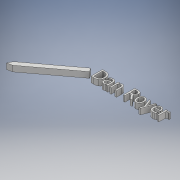
# Autodesk Inventor part: dan2
Saved by Autodesk Inventor 2017 (Build 210142000, 142)
## iProperties
Created: 2021-02-26
Part Number: dan2
Material: Generic
Document SubType Name: Modeling
Designer: paulg
Density: 1 g/cm^3
Appearance: Default
Author: paulg
Autodesk Inventor part; units mm, degrees
ref_plane "YZ Plane" through (0, 0, 0) normal (1, 0, 0) x (0, 1, 0)
ref_plane "XZ Plane" through (0, 0, 0) normal (0, 1, 0) x (-1, 0, 0)
ref_plane "XY Plane" through (0, 0, 0) normal (0, 0, 1) x (1, 0, 0)
sketch "Sketch1" plane through (0, 0, 0) normal (0, 0, 1) x (1, 0, 0)
  line L0 (-0.0217, 0.1086) -> (142.61, 0.1086) construction
  line L1 (142.61, 0.1086) -> (142.61, -1.7562) construction
  line L2 (142.61, -1.7562) -> (-0.0217, -1.7562) construction
  line L3 (-0.0217, -1.7562) -> (-0.0217, 0.1086) construction
  line L4 (-41.7116, -36.1087) -> (-2.9577, -7.16)
  line L5 (-2.9577, -7.16) -> (-5.3043, -4.0186)
  line L6 (-5.3043, -4.0186) -> (-44.0582, -32.9673)
  line L7 (-44.0582, -32.9673) -> (-41.7116, -36.1087)
  line L8 (-41.7116, -36.1087) -> (-5.3043, -4.0186) construction
  line L9 (-2.9577, -7.16) -> (-44.0582, -32.9673) construction
  line L10 (-44.0582, -32.9673) -> (-46.1916, -37.008)
  line L11 (-46.1916, -37.008) -> (-41.7116, -36.1087)
  line L12 (-46.1916, -37.008) -> (-42.8849, -34.538) construction
  spline S0 degree 2 poles (8.8762, -4.8995) (8.8762, -6.269) (7.766, -8.4732) (6.834, -9.0891) knots 0 0 0 1 2 2 2
  spline S1 degree 2 poles (6.834, -9.0891) (6.0723, -9.5672) (4.5083, -9.8914) (3.2927, -9.8914) knots 0 0 0 1 2 2 2
  line L13 (3.2927, -9.8914) -> (0.9912, -9.8914)
  line L14 (0.9912, -9.8914) -> (0.9912, 0.1086)
  line L15 (0.9912, 0.1086) -> (3.2684, 0.1086)
  spline S2 degree 2 poles (3.2684, 0.1086) (4.6784, 0.1086) (6.283, -0.3127) (6.8502, -0.6855) knots 0 0 0 1 2 2 2
  spline S3 degree 2 poles (6.8502, -0.6855) (7.8146, -1.3257) (8.8762, -3.4408) (8.8762, -4.8995) knots 0 0 0 1 2 2 2
  spline S4 degree 2 poles (7.4904, -4.8833) (7.4904, -3.7325) (6.7287, -2.1037) (5.975, -1.6418) knots 0 0 0 1 2 2 2
  spline S5 degree 2 poles (5.975, -1.6418) (5.4402, -1.3257) (4.2327, -1.0421) (3.3332, -1.0421) knots 0 0 0 1 2 2 2
  line L16 (3.3332, -1.0421) -> (2.3202, -1.0421)
  line L17 (2.3202, -1.0421) -> (2.3202, -8.7406)
  line L18 (2.3202, -8.7406) -> (3.3332, -8.7406)
  spline S6 degree 2 poles (3.3332, -8.7406) (4.2165, -8.7406) (5.5536, -8.457) (6.0966, -8.0761) knots 0 0 0 1 2 2 2
  spline S7 degree 2 poles (6.0966, -8.0761) (6.7935, -7.6061) (7.4904, -6.0502) (7.4904, -4.8833) knots 0 0 0 1 2 2 2
  spline S8 degree 2 poles (14.4029, -9.0972) (14.2489, -9.2106) (13.7303, -9.6158) (13.4872, -9.7374) knots 0 0 0 1 2 2 2
  spline S9 degree 2 poles (13.4872, -9.7374) (13.1549, -9.9157) (12.5309, -10.1021) (11.9637, -10.1021) knots 0 0 0 1 2 2 2
  spline S10 degree 2 poles (11.9637, -10.1021) (11.5018, -10.1021) (10.6671, -9.7536) (10.351, -9.4375) knots 0 0 0 1 2 2 2
  spline S11 degree 2 poles (10.351, -9.4375) (10.0512, -9.1296) (9.6865, -8.222) (9.6865, -7.7196) knots 0 0 0 1 2 2 2
  spline S12 degree 2 poles (9.6865, -7.7196) (9.6865, -6.9416) (10.3429, -5.8395) (11.0561, -5.5234) knots 0 0 0 1 2 2 2
  spline S13 degree 2 poles (11.0561, -5.5234) (11.6882, -5.2317) (13.4061, -5.0129) (14.4029, -4.9562) knots 0 0 0 1 2 2 2
  line L19 (14.4029, -4.9562) -> (14.4029, -4.7131)
  spline S14 degree 2 poles (14.4029, -4.7131) (14.4029, -4.2755) (14.1355, -3.7325) (13.8924, -3.5786) knots 0 0 0 1 2 2 2
  spline S15 degree 2 poles (13.8924, -3.5786) (13.6493, -3.4246) (12.9523, -3.3273) (12.5796, -3.3273) knots 0 0 0 1 2 2 2
  spline S16 degree 2 poles (12.5796, -3.3273) (12.142, -3.3273) (10.9588, -3.5867) (10.3672, -3.8379) knots 0 0 0 1 2 2 2
  line L20 (10.3672, -3.8379) -> (10.2943, -3.8379)
  line L21 (10.2943, -3.8379) -> (10.2943, -2.5494)
  spline S17 degree 2 poles (10.2943, -2.5494) (10.6428, -2.4521) (11.9475, -2.209) (12.5877, -2.209) knots 0 0 0 1 2 2 2
  spline S18 degree 2 poles (12.5877, -2.209) (13.3656, -2.209) (14.4272, -2.4521) (14.8486, -2.7682) knots 0 0 0 1 2 2 2
  spline S19 degree 2 poles (14.8486, -2.7682) (15.2619, -3.0761) (15.6671, -4.0567) (15.6671, -4.7617) knots 0 0 0 1 2 2 2
  line L22 (15.6671, -4.7617) -> (15.6671, -9.8914)
  line L23 (15.6671, -9.8914) -> (14.4029, -9.8914)
  line L24 (14.4029, -9.8914) -> (14.4029, -9.0972)
  line L25 (14.4029, -8.0437) -> (14.4029, -5.961)
  spline S20 degree 2 poles (14.4029, -5.961) (13.9491, -6.0016) (12.5796, -6.1393) (12.1501, -6.269) knots 0 0 0 1 2 2 2
  spline S21 degree 2 poles (12.1501, -6.269) (11.6476, -6.423) (10.9912, -7.0632) (10.9912, -7.6304) knots 0 0 0 1 2 2 2
  spline S22 degree 2 poles (10.9912, -7.6304) (10.9912, -8.2787) (11.7206, -8.9351) (12.4175, -8.9351) knots 0 0 0 1 2 2 2
  spline S23 degree 2 poles (12.4175, -8.9351) (13.0091, -8.9351) (13.9815, -8.4246) (14.4029, -8.0437) knots 0 0 0 1 2 2 2
  line L26 (23.3332, -9.8914) -> (22.069, -9.8914)
  line L27 (22.069, -9.8914) -> (22.069, -5.6126)
  spline S24 degree 2 poles (22.069, -5.6126) (22.069, -5.0939) (21.9718, -4.2025) (21.8259, -3.9351) knots 0 0 0 1 2 2 2
  spline S25 degree 2 poles (21.8259, -3.9351) (21.672, -3.6515) (21.1209, -3.376) (20.6509, -3.376) knots 0 0 0 1 2 2 2
  spline S26 degree 2 poles (20.6509, -3.376) (20.1809, -3.376) (19.1841, -3.8784) (18.706, -4.2836) knots 0 0 0 1 2 2 2
  line L28 (18.706, -4.2836) -> (18.706, -9.8914)
  line L29 (18.706, -9.8914) -> (17.4418, -9.8914)
  line L30 (17.4418, -9.8914) -> (17.4418, -2.3873)
  line L31 (17.4418, -2.3873) -> (18.706, -2.3873)
  line L32 (18.706, -2.3873) -> (18.706, -3.222)
  spline S27 degree 2 poles (18.706, -3.222) (19.2732, -2.7115) (20.3672, -2.1766) (20.9831, -2.1766) knots 0 0 0 1 2 2 2
  spline S28 degree 2 poles (20.9831, -2.1766) (22.0852, -2.1766) (23.3332, -3.6353) (23.3332, -5.021) knots 0 0 0 1 2 2 2
  line L33 (23.3332, -5.021) -> (23.3332, -9.8914)
  line L34 (37.2392, -9.8914) -> (35.5131, -9.8914)
  line L35 (35.5131, -9.8914) -> (32.3527, -5.9124)
  line L36 (32.3527, -5.9124) -> (30.8292, -5.9124)
  line L37 (30.8292, -5.9124) -> (30.8292, -9.8914)
  line L38 (30.8292, -9.8914) -> (29.5002, -9.8914)
  line L39 (29.5002, -9.8914) -> (29.5002, 0.1086)
  line L40 (29.5002, 0.1086) -> (32.0771, 0.1086)
  spline S29 degree 2 poles (32.0771, 0.1086) (32.9361, 0.1086) (34.095, -0.0777) (34.6217, -0.4181) knots 0 0 0 1 2 2 2
  spline S30 degree 2 poles (34.6217, -0.4181) (35.1484, -0.7585) (35.7562, -1.82) (35.7562, -2.6061) knots 0 0 0 1 2 2 2
  spline S31 degree 2 poles (35.7562, -2.6061) (35.7562, -3.7001) (34.6379, -5.1831) (33.6817, -5.5397) knots 0 0 0 1 2 2 2
  line L41 (33.6817, -5.5397) -> (37.2392, -9.8914)
  spline S32 degree 2 poles (34.3705, -2.7115) (34.3705, -2.2739) (34.0625, -1.6012) (33.7384, -1.3824) knots 0 0 0 1 2 2 2
  spline S33 degree 2 poles (33.7384, -1.3824) (33.4548, -1.1961) (32.7011, -1.0421) (32.1501, -1.0421) knots 0 0 0 1 2 2 2
  line L42 (32.1501, -1.0421) -> (30.8292, -1.0421)
  line L43 (30.8292, -1.0421) -> (30.8292, -4.8022)
  line L44 (30.8292, -4.8022) -> (31.9961, -4.8022)
  spline S34 degree 2 poles (31.9961, -4.8022) (32.5715, -4.8022) (33.4872, -4.5996) (33.8032, -4.2836) knots 0 0 0 1 2 2 2
  spline S35 degree 2 poles (33.8032, -4.2836) (34.095, -4.008) (34.3705, -3.2301) (34.3705, -2.7115) knots 0 0 0 1 2 2 2
  spline S36 degree 2 poles (44.1031, -6.1393) (44.1031, -8.0356) (42.2797, -10.1021) (40.7562, -10.1021) knots 0 0 0 1 2 2 2
  spline S37 degree 2 poles (40.7562, -10.1021) (39.1922, -10.1021) (37.4013, -7.9708) (37.4013, -6.1393) knots 0 0 0 1 2 2 2
  spline S38 degree 2 poles (37.4013, -6.1393) (37.4013, -4.2593) (39.2489, -2.1766) (40.7562, -2.1766) knots 0 0 0 1 2 2 2
  spline S39 degree 2 poles (40.7562, -2.1766) (42.2797, -2.1766) (44.1031, -4.2512) (44.1031, -6.1393) knots 0 0 0 1 2 2 2
  spline S40 degree 2 poles (42.7984, -6.1393) (42.7984, -4.6807) (41.7368, -3.2625) (40.7562, -3.2625) knots 0 0 0 1 2 2 2
  spline S41 degree 2 poles (40.7562, -3.2625) (39.7757, -3.2625) (38.706, -4.6807) (38.706, -6.1393) knots 0 0 0 1 2 2 2
  spline S42 degree 2 poles (38.706, -6.1393) (38.706, -7.5575) (39.7757, -9.0162) (40.7562, -9.0162) knots 0 0 0 1 2 2 2
  spline S43 degree 2 poles (40.7562, -9.0162) (41.7287, -9.0162) (42.7984, -7.5818) (42.7984, -6.1393) knots 0 0 0 1 2 2 2
  line L45 (51.2911, -2.3873) -> (47.2554, -12.6547)
  line L46 (47.2554, -12.6547) -> (45.9021, -12.6547)
  line L47 (45.9021, -12.6547) -> (47.2473, -9.5267)
  line L48 (47.2473, -9.5267) -> (44.5245, -2.3873)
  line L49 (44.5245, -2.3873) -> (45.8859, -2.3873)
  line L50 (45.8859, -2.3873) -> (47.9361, -7.9465)
  line L51 (47.9361, -7.9465) -> (49.9783, -2.3873)
  line L52 (49.9783, -2.3873) -> (51.2911, -2.3873)
  spline S44 degree 2 poles (55.505, -10.0615) (53.706, -10.0615) (51.7287, -8.0437) (51.7287, -6.1798) knots 0 0 0 1 2 2 2
  spline S45 degree 2 poles (51.7287, -6.1798) (51.7287, -4.3484) (53.6493, -2.1766) (55.1971, -2.1766) knots 0 0 0 1 2 2 2
  spline S46 degree 2 poles (55.1971, -2.1766) (55.894, -2.1766) (56.9718, -2.5818) (57.3689, -3.0113) knots 0 0 0 1 2 2 2
  spline S47 degree 2 poles (57.3689, -3.0113) (57.7741, -3.4408) (58.2036, -4.6807) (58.2036, -5.5802) knots 0 0 0 1 2 2 2
  line L53 (58.2036, -5.5802) -> (58.2036, -6.269)
  line L54 (58.2036, -6.269) -> (53.0091, -6.269)
  spline S48 degree 2 poles (53.0091, -6.269) (53.0091, -7.5737) (54.3219, -8.9594) (55.4888, -8.9594) knots 0 0 0 1 2 2 2
  spline S49 degree 2 poles (55.4888, -8.9594) (55.9021, -8.9594) (56.7044, -8.773) (57.0285, -8.6272) knots 0 0 0 1 2 2 2
  spline S50 degree 2 poles (57.0285, -8.6272) (57.3689, -8.4651) (57.8389, -8.1815) (57.9929, -8.0518) knots 0 0 0 1 2 2 2
  line L55 (57.9929, -8.0518) -> (58.0658, -8.0518)
  line L56 (58.0658, -8.0518) -> (58.0658, -9.4294)
  spline S51 degree 2 poles (58.0658, -9.4294) (57.847, -9.5186) (57.1825, -9.7779) (56.9232, -9.8508) knots 0 0 0 1 2 2 2
  spline S52 degree 2 poles (56.9232, -9.8508) (56.5585, -9.9562) (55.9588, -10.0615) (55.505, -10.0615) knots 0 0 0 1 2 2 2
  spline S53 degree 2 poles (56.9718, -5.3046) (56.9556, -4.7941) (56.7449, -4.0486) (56.5423, -3.7974) knots 0 0 0 1 2 2 2
  spline S54 degree 2 poles (56.5423, -3.7974) (56.3235, -3.5137) (55.6347, -3.2139) (55.1241, -3.2139) knots 0 0 0 1 2 2 2
  spline S55 degree 2 poles (55.1241, -3.2139) (54.6217, -3.2139) (53.9167, -3.5137) (53.6249, -3.8055) knots 0 0 0 1 2 2 2
  spline S56 degree 2 poles (53.6249, -3.8055) (53.3413, -4.1053) (53.0496, -4.8265) (53.0091, -5.3046) knots 0 0 0 1 2 2 2
  line L57 (53.0091, -5.3046) -> (56.9718, -5.3046)
  line L58 (63.4629, -3.7406) -> (63.398, -3.7406)
  spline S57 degree 2 poles (63.398, -3.7406) (63.2522, -3.7001) (62.9361, -3.6839) (62.7173, -3.6839) knots 0 0 0 1 2 2 2
  spline S58 degree 2 poles (62.7173, -3.6839) (62.2068, -3.6839) (61.2019, -4.1296) (60.7481, -4.5672) knots 0 0 0 1 2 2 2
  line L59 (60.7481, -4.5672) -> (60.7481, -9.8914)
  line L60 (60.7481, -9.8914) -> (59.4839, -9.8914)
  line L61 (59.4839, -9.8914) -> (59.4839, -2.3873)
  line L62 (59.4839, -2.3873) -> (60.7481, -2.3873)
  line L63 (60.7481, -2.3873) -> (60.7481, -3.5056)
  spline S59 degree 2 poles (60.7481, -3.5056) (61.4369, -2.8897) (62.4661, -2.3873) (62.9523, -2.3873) knots 0 0 0 1 2 2 2
  spline S60 degree 2 poles (62.9523, -2.3873) (63.1468, -2.3873) (63.3413, -2.4035) (63.4629, -2.4278) knots 0 0 0 1 2 2 2
  line L64 (63.4629, -2.4278) -> (63.4629, -3.7406)
  point P0 (0, 0)
  point P1 (-23.5079, -20.0636)
  constraints: 18 end point, 3 midpoint, 3 parallel, 1 perpendicular, 2 other
extrude "Extrusion1" add sketch "Sketch1" along normal blind 5
body "Solid1"
